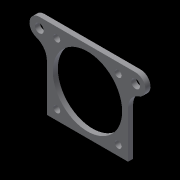
# Autodesk Inventor part: FanMount
Saved by Autodesk Inventor 2014 (Build 180170000, 170)
## iProperties
Created: 2015-07-08
Part Number: FanMount
Material: Generic
Document SubType Name: Modeling
Designer: Scott
Density: 1 g/cm^3
Appearance: Default
Author: Scott
Autodesk Inventor part; units mm, degrees
ref_plane "YZ Plane" through (0, 0, 0) normal (1, 0, 0) x (0, 1, 0)
ref_plane "XZ Plane" through (0, 0, 0) normal (0, 1, 0) x (-1, 0, 0)
ref_plane "XY Plane" through (0, 0, 0) normal (0, 0, 1) x (1, 0, 0)
sketch "Sketch1" plane through (0, 0, 0) normal (0, 0, 1) x (1, 0, 0)
  line L0 (0, 0) -> (41, 0)
  line L1 (41, 0) -> (41, 41)
  line L2 (41, 41) -> (0, 41)
  line L3 (0, 41) -> (0, 0)
  line L4 (20.5, 20.5) -> (20.5, 36)
  line L5 (20.5, 36) -> (5, 36)
  circle A0 centre (5, 36) radius 1.725
  circle A1 centre (36, 36) radius 1.725
  circle A2 centre (5, 5) radius 1.725
  circle A3 centre (36, 5) radius 1.725
  circle A4 centre (20.5, 20.5) radius 17.5
  line L6 (0, 36) -> (-3.81, 36)
  circle A5 centre (-3.81, 36) radius 2.2225
  line L7 (41, 36) -> (44.81, 36)
  circle A6 centre (44.81, 36) radius 2.2225
  line L8 (0, 41) -> (-3.81, 41)
  line L9 (0, 36) -> (0, 30.9962)
  line L10 (0, 30.9962) -> (-3.81, 30.9962)
  arc A7 (-3.81, 41) -> (-3.81, 30.9962) centre (-3.81, 35.9981) ccw
  line L11 (41, 41) -> (44.81, 41)
  line L12 (41, 36) -> (41, 30.9962)
  line L13 (41, 30.9962) -> (44.81, 30.9962)
  arc A8 (44.81, 30.9962) -> (44.81, 41) centre (44.81, 35.9981) ccw
  dimension "d0" = 41
  dimension "d1" = 41
  dimension "d2" = 15.5
  dimension "d3" = 15.5
  dimension "d4" = 3.45
  dimension "d7" = 31
  dimension "d10" = 31
  dimension "d13" = 35
  dimension "d14" = 3.81
  dimension "d15" = 4.445
  dimension "d16" = 3.81
  dimension "d17" = 4.445
  dimension "d18" = 5.0038
  dimension "d19" = 5.0038
  constraints: 28 end point, 9 centre point, 5 perpendicular, 4 coincident, 4 parallel, 4 point on circle, 4 point on line, 4 tangent, 2 collinear, 2 horizontal, 1 vertical, 6 other
  measures "d0" distance of L2.end L1.end
  measures "d1" distance of L1.end L0.end
  measures "d2" distance of L4.start L4.end
  measures "d3" distance of L4.end L5.end
  measures "d4" diameter of A0
  measures "d7" distance of A0.centre A1.centre
  measures "d10" distance of A0.centre A2.centre
  measures "d13" diameter of A4
  measures "d14" distance of L6.start L6.end
  measures "d15" diameter of A5
  measures "d16" distance of L7.start L7.end
  measures "d17" diameter of A6
  measures "d18" distance of L6.start L9.end
  measures "d19" distance of L7.start L12.end
extrude "Extrusion1" add sketch "Sketch1" along normal blind 2.54
fillet "Fillet1" radius 7.9375 2 edges at (0, 30.9962, 1.27) (41, 30.9962, 1.27)
body "Solid1"
